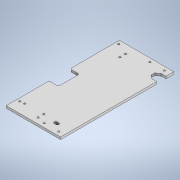
# Autodesk Inventor part: Battery Side Plate
Saved by Autodesk Inventor 2021 (Build 250183000, 183)
## iProperties
Created: 2020-07-17
Part Number: Battery Side Plate
Material: Generic
Document SubType Name: Modeling
Designer: jgray
Density: 1 g/cm^3
Appearance: Default
Author: jgray
Autodesk Inventor part; units mm, degrees
ref_plane "YZ Plane" through (0, 0, 0) normal (1, 0, 0) x (0, 1, 0)
ref_plane "XZ Plane" through (0, 0, 0) normal (0, 1, 0) x (-1, 0, 0)
ref_plane "XY Plane" through (0, 0, 0) normal (0, 0, 1) x (1, 0, 0)
sketch "Sketch1" plane through (0, 0, 0) normal (0, 1, 0) x (-1, 0, 0)
  line L0 (0, 0) -> (116.2, 0)
  line L1 (116.2, 0) -> (116.2, -242)
  line L2 (116.2, -242) -> (0, -242)
  line L3 (0, -242) -> (0, 0)
  dimension "d0" = 116.2
  dimension "d1" = 242
  constraints: 8 end point, 2 parallel, 1 horizontal, 1 perpendicular
  measures "d0" distance of L1.end L2.end
  measures "d1" distance of L0.end L1.end
extrude "Extrusion1" add sketch "Sketch1" along normal blind 5
sketch "Sketch2" plane through (0, 5, 0) normal (0, 1, 0) x (1, 0, 0)
  line L0 (-43, 8) -> (-12, 8) construction
  line L1 (-12, 8) -> (-12, 234) construction
  line L2 (-12, 234) -> (-43, 234) construction
  line L3 (-43, 234) -> (-43, 8) construction
  line L4 (-116.2, 0) -> (0, 0) construction
  line L5 (0, 242) -> (-116.2, 242) construction
  line L6 (0, 0) -> (0, 242) construction
  dimension "d4" = 8
  dimension "d5" = 8
  dimension "d6" = 12
  dimension "d7" = 31
  constraints: 8 end point, 4 coincident, 2 parallel, 1 horizontal, 1 perpendicular
  measures "d4" distance between parallel lines of L4 L0
  measures "d5" distance between parallel lines of L5 L2
  measures "d6" distance between parallel lines of L6 L1
  measures "d7" distance of L0.start L0.end
hole "Hole1" at (-12, 5, -8) at (-43, 5, -8) at (-43, 5, -234) at (-12, 5, -234) direction (0, -1, 0) diameter 3.8 end through all
sketch "Sketch3" plane through (0, 5, 0) normal (0, 1, 0) x (1, 0, 0)
  line L0 (-128.5064, 215.5) -> (22.7754, 215.5) construction
  line L1 (0, 242) -> (-116.2, 242) projected
  line L2 (0, 225.5) -> (-18, 225.5)
  line L3 (-18, 225.5) -> (-18, 205.5)
  line L4 (-18, 205.5) -> (0, 205.5)
  line L5 (0, 205.5) -> (0, 225.5)
  line L6 (0, 225.5) -> (-18, 205.5) construction
  line L7 (-18, 225.5) -> (0, 205.5) construction
  line L8 (0, 0) -> (0, 242) projected
  line L9 (-18, 211.5) -> (-10, 205.5)
  line L10 (-18, 219.5) -> (-10, 225.5)
  point P0 (-9, 215.5)
  point P1 (-18, 215.5)
  dimension "d15" = 26.5
  dimension "d16" = 20
  dimension "d17" = 18
  dimension "d18" = 8
  dimension "d19" = 10
  constraints: 18 end point, 4 point on line, 3 midpoint, 2 parallel, 2 symmetric about line, 1 collinear, 1 horizontal, 1 perpendicular
  measures "d15" distance between parallel lines of L0 L1
  measures "d16" distance of L3.end L2.end
  measures "d17" distance between parallel lines of L5 L3
  measures "d18" diameter of L9.start L0
  measures "d19" distance of L4.end L9.end
extrude "Extrusion2" cut sketch "Sketch3" against normal through all contours L5 L4 L9 L3 L10 L2
fillet "Fillet1" radius 2 4 edges at (-18, 2.5, -219.5) (-10, 2.5, -225.5) (-18, 2.5, -211.5) (-10, 2.5, -205.5)
sketch "Sketch4" plane through (0, 5, 0) normal (0, 1, 0) x (1, 0, 0)
  line L0 (-84.2, 269.0758) -> (-84.2, -69.3617) construction
  line L1 (0, 0) -> (0, 205.5) construction
  line L2 (-116.2, 0) -> (0, 0) construction
  line L3 (0, 242) -> (-116.2, 242) construction
  line L4 (-116.2, 242) -> (-116.2, 0) projected
  line L5 (-60, 78.142) -> (-60, -51.5949) construction
  point P0 (-84.2, 223)
  point P1 (-84.2, 211)
  point P2 (-60, 24)
  point P3 (-60, 12)
  dimension "d24" = 12
  dimension "d25" = 12
  dimension "d26" = 12
  dimension "d27" = 31
  dimension "d35" = 32
  dimension "d36" = 60
  constraints: 4 end point, 4 point on line, 2 vertical
  measures "d24" distance of point (-60, 12) point (-60, 24)
  measures "d25" distance from line of L2 point (-60, 12)
  measures "d26" distance of point (-84.2, 211) point (-84.2, 223)
  measures "d27" distance from line of point (-84.2, 211) L3
  measures "d35" distance between parallel lines of L4 L0
  measures "d36" distance between parallel lines of L1 L5
hole "Hole2" at (-84.2, 5, -223) at (-84.2, 5, -211) at (-60, 5, -24) at (-60, 5, -12) direction (0, -1, 0) diameter 3.8 end through all
sketch "Sketch5" plane through (0, 5, 0) normal (0, 1, 0) x (1, 0, 0)
  line L0 (-116.2, 242) -> (-116.2, 0) projected
  line L1 (-116.2, 0) -> (0, 0) projected
  point P0 (-100.2, 23.25)
  dimension "d37" = 16
  dimension "d38" = 23.25
  measures "d37" distance from line of point (-100.2, 23.25) L0
  measures "d38" distance from line of L1 point (-100.2, 23.25)
hole "Hole3" at (-100.2, 5, -23.25) direction (0, -1, 0) diameter 3.8 end through all
sketch "Sketch6" plane through (0, 5, 0) normal (0, 1, 0) x (1, 0, 0)
  line L0 (-109.7, 280.0258) -> (-109.7, -41.1522) construction
  line L1 (-116.2, 242) -> (-116.2, 0) projected
  line L2 (0, 242) -> (-116.2, 242) projected
  point P0 (0, 0)
  point P1 (-109.7, 234)
  point P2 (-109.7, 22.25)
  dimension "d46" = 6.5
  dimension "d47" = 8
  dimension "d48" = 211.75
  constraints: 2 end point, 2 point on line, 1 vertical
  measures "d46" distance between parallel lines of L1 L0
  measures "d47" distance from line of point (-109.7, 234) L2
  measures "d48" distance of point (-109.7, 22.25) point (-109.7, 234)
hole "Hole4" at (-109.7, 5, -234) at (-109.7, 5, -22.25) direction (0, -1, 0) diameter 3.8 end through all
sketch "Sketch7" plane through (0, 5, 0) normal (0, 1, 0) x (1, 0, 0)
  line L0 (-50.7253, 21) -> (31.7934, 21) construction
  line L1 (-116.2, 0) -> (0, 0) construction
  line L2 (-32, 24) -> (-27.5, 24)
  line L3 (-25, 21.5) -> (-25, 20.5)
  line L4 (-27.5, 18) -> (-32, 18)
  line L5 (-32, 18) -> (-32, 21)
  line L6 (-32, 24) -> (-25, 18) construction
  line L7 (-25, 24) -> (-32, 18) construction
  line L8 (0, 0) -> (0, 205.5) construction
  arc A0 (-32, 24) -> (-32, 18) centre (-32, 21) ccw
  arc A1 (-25, 21.5) -> (-27.5, 24) centre (-27.5, 21.5) ccw
  arc A2 (-27.5, 18) -> (-25, 20.5) centre (-27.5, 20.5) ccw
  point P0 (-28.5, 21)
  dimension "d56" = 21
  dimension "d57" = 7
  dimension "d58" = 6
  dimension "d59" = 25
  dimension "d62" = 2.5
  constraints: 14 end point, 6 point on circle, 6 point on line, 4 tangent, 3 centre point, 2 horizontal, 2 midpoint, 2 parallel, 1 equal radius, 1 perpendicular
  measures "d56" distance between parallel lines of L1 L0
  measures "d57" distance of L4.end L6.end
  measures "d58" distance of L7.start L6.end
  measures "d59" distance between parallel lines of L8 L3
  measures "d62" radius of A1
extrude "Extrusion3" cut sketch "Sketch7" against normal blind 10
sketch "Sketch8" plane through (0, 5, 0) normal (0, 1, 0) x (1, 0, 0)
  line L0 (-195.7233, 114) -> (78.1714, 114) construction
  line L1 (-116.2, 0) -> (0, 0) projected
  line L2 (-136.2, 91.5) -> (-96.2, 91.5)
  line L3 (-96.2, 91.5) -> (-96.2, 136.5)
  line L4 (-96.2, 136.5) -> (-136.2, 136.5)
  line L5 (-136.2, 136.5) -> (-136.2, 91.5)
  line L6 (-116.2, 242) -> (-116.2, 0) projected
  line L7 (-136.2, 91.5) -> (-96.2, 136.5) construction
  line L8 (-96.2, 91.5) -> (-136.2, 136.5) construction
  point P0 (-116.2, 114)
  point P1 (-116.2, 136.5)
  point P2 (-116.2, 91.5)
  dimension "d63" = 114
  dimension "d64" = 40
  dimension "d65" = 45
  constraints: 14 end point, 2 horizontal, 2 midpoint, 2 parallel, 2 point on line, 1 perpendicular
  measures "d63" distance between parallel lines of L1 L0
  measures "d64" distance of L4.end L3.end
  measures "d65" distance of L3.end L2.end
extrude "Extrusion4" cut sketch "Sketch8" against normal through all contours L6 L4 L3 L2
fillet "Fillet2" radius 4 4 edges at (-116.2, 2.5, -136.5) (-116.2, 2.5, -91.5) (-96.2, 2.5, -91.5) (-96.2, 2.5, -136.5)
fillet "Fillet3" radius 2 1 edges at (-116.2, 2.5, -242)
body "Solid1"
